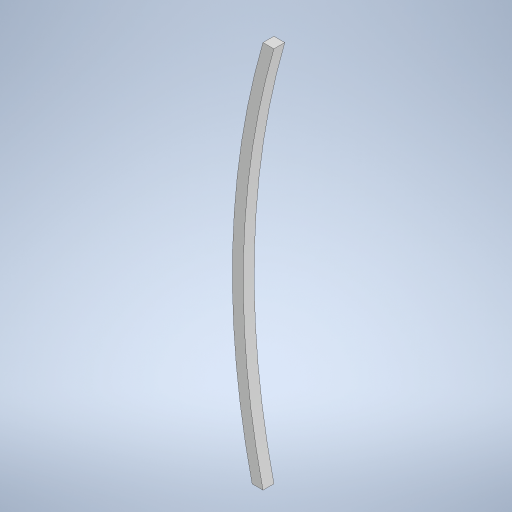
# Autodesk Inventor part: ferris_wheel_outer_ring
Saved by Autodesk Inventor 2023 (Build 270158000, 158)
## iProperties
Created: 2025-10-20
Part Number: ferris_wheel_outer_ring
Material: Generic
Document SubType Name: Modeling
Designer: Justin Pascual
Density: 1 g/cm^3
Appearance: Default
Author: Justin Pascual
Autodesk Inventor part; units mm, degrees
ref_plane "YZ Plane" through (0, 0, 0) normal (1, 0, 0) x (0, 1, 0)
ref_plane "XY Plane" through (0, 0, 0) normal (0, 0, 1) x (1, 0, 0)
sketch "Sketch2" plane through (0, 0, 0) normal (0, 1, 0) x (-1, 0, 0)
  line L0 (0, 0) -> (-3.81, 0)
  line L1 (-3.81, 0) -> (-3.81, -3.81)
  line L2 (-3.81, -3.81) -> (0, -3.81)
  line L3 (0, -3.81) -> (0, 0)
  dimension "d4" = 3.81
  dimension "d5" = 3.81
  constraints: 8 end point, 2 parallel, 1 horizontal, 1 perpendicular
  measures "d4" distance of L2.end L1.end
  measures "d5" distance of L1.end L0.end
ref_plane "Work Plane1" through (0, 131.826, 0) normal (0, 1, 0) x (-1, 0, 0)
sketch "Sketch3" plane through (0, 131.826, 0) normal (0, 1, 0) x (-1, 0, 0)
  line L0 (-3.81, -3.81) -> (0, -3.81) projected
  line L1 (0, -3.81) -> (0, 0) construction
  line L2 (-3.81, 0) -> (-3.81, -3.81) construction
  line L3 (0, 0) -> (-3.81, 0) construction
  line L4 (-3.81, -3.81) -> (0, -3.81)
  line L5 (0, -3.81) -> (0, -7.62)
  line L6 (0, -7.62) -> (-3.81, -7.62)
  line L7 (-3.81, -7.62) -> (-3.81, -3.81)
  dimension "d7" = 3.81
  dimension "d8" = 3.81
  constraints: 8 end point, 2 parallel, 1 horizontal, 1 perpendicular
  measures "d7" distance of L5.end L6.end
  measures "d8" distance of L4.end L5.end
ref_plane "Work Plane2" through (3.81, 0, -3.81) normal (0, -0.0288897, -0.9995826) x (-1, 0, 0)
sketch "Sketch4" plane through (3.81, 0, -3.81) normal (0, -0.0288897, -0.9995826) x (-1, 0, 0)
  circle A0 centre (249.1014, 65.9405) radius 254 construction
  line L0 (3.81, 0) -> (3.81, 131.881) construction
  arc A1 (3.81, 0) -> (3.81, 131.881) centre (-241.4814, 65.9405) ccw
  point P0 (3.81, -0.1101)
  dimension "d9" = 508
  constraints: 4 point on circle, 2 centre point, 2 end point, 1 symmetric about line, 1 vertical
  measures "d9" diameter of A0
sweep "Sweep1" add profiles "Sketch2" path "Sketch4" keep normal constant yes
body "Solid2"
